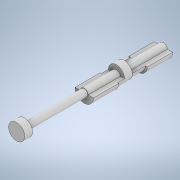
# Autodesk Inventor part: балансирный_вал
Saved by Autodesk Inventor 2021 (Build 250183000, 183)
## iProperties
Created: 2021-06-15
Part Number: балансирный_вал
Material: Типовые
Document SubType Name: Modeling
Designer: panda
Density: 1 g/cm^3
Appearance: По умолчанию
Author: panda
Autodesk Inventor part; units mm, degrees
ref_plane "YZ Plane" through (0, 0, 0) normal (1, 0, 0) x (0, 1, 0)
ref_plane "XZ Plane" through (0, 0, 0) normal (0, 1, 0) x (-1, 0, 0)
ref_plane "XY Plane" through (0, 0, 0) normal (0, 0, 1) x (1, 0, 0)
sketch "Эскиз1" plane through (0, 0, 0) normal (0, 0, 1) x (1, 0, 0)
  arc A0 (-20, 0) -> (20, 0) centre (0, 0) ccw
  line L0 (-20, 0) -> (20, 0)
  circle A1 centre (0, 0) radius 8.5
  point P0 (8.5, 0)
  point P1 (-8.5, 0)
  dimension "d0" = 40
  dimension "d1" = 17
  constraints: 2 centre point, 2 coincident, 2 end point, 2 point on circle, 1 horizontal
  measures "d0" diameter of A0
  measures "d1" diameter of A1
extrude "Выдавливание1" add sketch "Эскиз1" against normal blind 55
sketch "Эскиз2" plane through (0, 0, 0) normal (0, 0, 1) x (1, 0, 0)
  circle A0 centre (0, 0) radius 8.5
  circle A1 centre (0, 0) radius 16
  line L0 (-20, 0) -> (-8.5, 0) projected
  line L1 (-16, 0) -> (16, 0)
  point P0 (8.5, 0)
  point P1 (-8.5, 0)
  dimension "d4" = 32
  dimension "d10" = 17
  constraints: 2 centre point, 2 coincident, 2 end point, 2 point on circle, 1 collinear, 1 point on line
  measures "d4" diameter of A1
  measures "d10" diameter of A0
extrude "Выдавливание2" add sketch "Эскиз2" along normal blind 30 contours L1 A0 | L1 A1 L0 A0 | A0 L1 picked at (13.2627, -1.9544)
sketch "Эскиз3" plane through (0, 0, 30) normal (0, 0, 1) x (1, 0, 0)
  circle A0 centre (0, 0) radius 17.5
  dimension "d7" = 35
  constraints: 1 centre point, 1 coincident
  measures "d7" diameter of A0
extrude "Выдавливание3" add sketch "Эскиз3" along normal blind 17
sketch "Эскиз4" plane through (0, 0, 47) normal (0, 0, 1) x (1, 0, 0)
  circle A0 centre (0, 0) radius 8.5
  circle A1 centre (0, 0) radius 17.5
  line L0 (-16, 0) -> (-20, 0) projected
  line L1 (-17.5, 0) -> (17.5, 0)
  line L2 (8.5, 0) -> (20, 0) projected
  point P0 (-18, 0)
  point P1 (-8.5, 0)
  dimension "d25" = 17
  dimension "d22" = 35
  constraints: 2 end point, 2 point on circle, 1 centre point, 1 coincident, 1 collinear, 1 midpoint, 1 point on line, 2 other
  measures "d22" diameter of A1
extrude "Выдавливание4" add sketch "Эскиз4" along normal blind 15 contours L1 A0 | L1 A1 L0 A0 | A0 L1 picked at (14.2482, -2.0741)
sketch "Эскиз6" plane through (0, 0, 62) normal (0, 0, 1) x (1, 0, 0)
  circle A0 centre (0, 0) radius 8.5
  line L0 (-16, 0) -> (-20, 0) projected
  arc A1 (-20, 0) -> (20, 0) centre (0, 0) ccw projected
  line L1 (-20, 0) -> (20, 0)
  line L2 (8.5, 0) -> (20, 0) projected
  circle A2 centre (0, 0) radius 20
  line L3 (-20, 0) -> (-8.5, 0) projected
  line L4 (-20, 0) -> (20, 0)
  point P0 (-8.5, 0)
  dimension "d24" = 17
  constraints: 4 end point, 1 centre point, 1 coincident, 1 collinear, 1 horizontal, 1 horizontal alignment, 2 other
  measures "d24" diameter of A0
extrude "Выдавливание5" add sketch "Эскиз6" along normal blind 55 contours L1 A0 | L1 A1 L0 A0 | A0 L1
sketch "Эскиз7" plane through (0, 0, 117) normal (0, 0, 1) x (1, 0, 0)
  circle A0 centre (0, 0) radius 7.5
  dimension "d26" = 15
  constraints: 1 centre point, 1 coincident
  measures "d26" diameter of A0
extrude "Выдавливание6" add sketch "Эскиз7" along normal blind 130
sketch "Эскиз8" plane through (0, 0, 247) normal (0, 0, 1) x (1, 0, 0)
  circle A0 centre (0, 0) radius 17.5
  dimension "d23" = 35
  constraints: 1 centre point, 1 coincident
  measures "d23" diameter of A0
extrude "Выдавливание7" add sketch "Эскиз8" along normal blind 17
